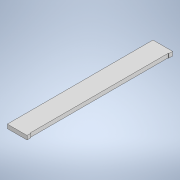
# Autodesk Inventor part: modelGateCover
Saved by Autodesk Inventor 2020 (Build 240168000, 168)
## iProperties
Created: 2023-11-14
Part Number: modelGateCover
Material: Generic
Document SubType Name: Sheet Metal
Designer: jirka
Density: 1 g/cm^3
Sheet Metal Rule: Default_mm
Appearance: Default
Author: jirka
Autodesk Inventor part; units mm, degrees
ref_plane "YZ Plane" through (0, 0, 0) normal (1, 0, 0) x (0, 1, 0)
ref_plane "XZ Plane" through (0, 0, 0) normal (0, 1, 0) x (-1, 0, 0)
ref_plane "XY Plane" through (0, 0, 0) normal (0, 0, 1) x (1, 0, 0)
sketch "Sketch1" plane through (0, 0, 0) normal (0, 1, 0) x (-1, 0, 0)
  line L0 (5, 37) -> (-5, 37)
  line L1 (-5, 37) -> (-5, -37)
  line L2 (-5, -37) -> (5, -37)
  line L3 (5, -37) -> (5, 37)
  point P0 (0, 0)
  dimension "d0" = 10
  dimension "d1" = 74
  dimension "d2" = 5
  dimension "d3" = 37
  constraints: 8 end point, 2 parallel, 1 horizontal, 1 perpendicular
  measures "d0" distance of L1.end L2.end
  measures "d1" distance of L0.end L1.end
  measures "d2" distance from line of L3 point (0, 0)
  measures "d3" distance from line of L2 point (0, 0)
extrude "Extrusion1" add sketch "Sketch1" along normal blind 2
sketch "Sketch2" plane through (5, 0, 37) normal (1, 0, 0) x (0, 0, -1)
  line L0 (74, 2) -> (0, 2) projected
  line L1 (74, 0) -> (0, 0) projected
  line L2 (0, 2) -> (2, 2)
  line L3 (2, 2) -> (2, 0)
  line L4 (2, 0) -> (0, 0)
  line L5 (0, 0) -> (0, 2)
  line L6 (2, 0) -> (74, 0)
  line L7 (74, 0) -> (74, 2)
  line L8 (74, 2) -> (2, 2)
  line L9 (2, 2) -> (2, 0)
  line L10 (74, 0) -> (72, 0)
  line L11 (72, 0) -> (72, 2)
  line L12 (72, 2) -> (74, 2)
  line L13 (74, 2) -> (74, 0)
  point P0 (37, 0)
  point P1 (2, 2)
  dimension "d6" = 72
  constraints: 24 end point, 6 parallel, 3 horizontal, 3 perpendicular, 3 point on line
  measures "d6" distance of L8.end L7.end
extrude "Extrusion2" cut sketch "Sketch2" against normal blind 0.3 contours L11 L1 L3 L0
equation "\"d2\" = 0.5 * d0"
equation "\"d3\" = 0.5 * d1"
equation "\"BendRadius\" = Thickness"
equation "\"BendReliefWidth\" = Thickness"
equation "\"BendReliefDepth\" = 0.5 * Thickness"
equation "\"CornerReliefSize\" = 4 * Thickness"
equation "\"MinimumRemnant\" = 2 * Thickness"
equation "\"TransitionRadius\" = BendRadius"
equation "\"JacobiRadiusSize\" = BendRadius"
equation "\"GapSize\" = Thickness"
equation "\"Thickness\" = 0.5"
body "Solid1"
